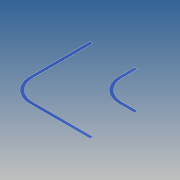
# Autodesk Inventor part: Bocht 90 graden
Saved by Autodesk Inventor 2020 (Build 240168000, 168)
## iProperties
Created: 2019-11-19
Part Number: Bocht 90 graden
Material: Generic
Document SubType Name: Modeling
Designer: Berkant
Density: 1 g/cm^3
Appearance: Default
Author: Berkant
Autodesk Inventor part; units mm, degrees
ref_plane "YZ Plane" through (0, 0, 0) normal (1, 0, 0) x (0, 1, 0)
ref_plane "XZ Plane" through (0, 0, 0) normal (0, 1, 0) x (-1, 0, 0)
ref_plane "XY Plane" through (0, 0, 0) normal (0, 0, 1) x (1, 0, 0)
sketch "Sketch1" plane through (0, 0, 0) normal (0, 1, 0) x (-1, 0, 0)
  arc A0 (200, 0) -> (0, 200) centre (0, 0) ccw
  line L0 (0, 200) -> (-200, 200)
  line L1 (200, 0) -> (200, -200)
  line L2 (0, 230) -> (-200, 230)
  line L3 (230, 0) -> (230, -200)
  arc A1 (230, 0) -> (0, 230) centre (0, 0) ccw
  arc A2 (200, 0) -> (0, 200) centre (0, 0) ccw
  line L4 (-200, -430) -> (-200, -580)
  line L5 (-200, 230) -> (-350, 230)
  line L6 (-350, 200) -> (-200, 200)
  line L7 (200, -200) -> (200, -380)
  line L8 (230, -380) -> (230, -200)
  line L9 (200, -380) -> (200, -580)
  line L10 (200, -580) -> (230, -580)
  line L11 (230, -580) -> (230, -380)
  line L12 (-200, -580) -> (-230, -580)
  line L13 (-230, -580) -> (-230, -430)
  arc A3 (-200, -430) -> (-430, -200) centre (-430, -430) ccw
  arc A4 (230, 0) -> (0, 230) centre (0, 0) ccw
  arc A5 (-230, -430) -> (-430, -230) centre (-430, -430) ccw
  line L14 (-430, -200) -> (-580, -200)
  line L15 (-580, -200) -> (-580, -230)
  line L16 (-580, -230) -> (-430, -230)
  line L17 (-350, 230) -> (-580, 230)
  line L18 (-580, 230) -> (-580, 200)
  line L19 (-580, 200) -> (-350, 200)
  dimension "d25" = 30
  dimension "d26" = 150
  dimension "d27" = 400
  dimension "d28" = 400
  constraints: 40 end point, 12 point on circle, 11 horizontal, 11 vertical, 7 perpendicular, 6 centre point, 2 coincident, 1 collinear, 1 tangent, 21 other
  measures "d25" distance of L4.end L12.end
  measures "d26" distance of L14.start L14.end
  measures "d27" distance between parallel lines of L19 L14
  measures "d28" distance between parallel lines of L9 L4
extrude "Extrusion1" add sketch "Sketch1" along normal blind 0.5
body "Solid1"
